Autodesk Fusion 360 part; units mm, degrees
note: some values were not read from the file. Chosen so that the rebuilt part matches the saved one: which face or edge a step refers to. Set by a fixed rule: which sketch regions a step uses.
(part 3 of 3)
sketch "SecondHoles" plane through (0, 0, 0) normal (0, 0, 1) x (1, 0, 0)
  circle A0 centre (-16.518, 39.156) radius 0.5
  arc A1 (-17.021, 38.656) -> (-17.021, 39.656) centre (-17.018, 39.156) ccw
  circle A2 centre (-16.518, 36.656) radius 0.5
  circle A3 centre (-17.018, 36.656) radius 0.5
  circle A4 centre (-16.518, 34.156) radius 0.5
  circle A5 centre (-17.018, 34.156) radius 0.5
  circle A6 centre (-16.518, 31.656) radius 0.5
  circle A7 centre (-16.518, 29.156) radius 0.5
  arc A8 (-17.021, 28.656) -> (-17.021, 29.656) centre (-17.018, 29.156) ccw
  circle A9 centre (-16.518, 26.656) radius 0.5
  arc A10 (-16.718, 26.256) -> (-16.718, 27.056) centre (-17.018, 26.656) ccw
  circle A11 centre (-16.518, 24.156) radius 0.5
  arc A12 (-17.021, 23.656) -> (-17.021, 24.656) centre (-17.018, 24.156) ccw
  circle A13 centre (-16.518, 21.656) radius 0.5
  circle A14 centre (-16.518, 19.156) radius 0.5
  arc A15 (-17.021, 18.656) -> (-17.021, 19.656) centre (-17.018, 19.156) ccw
  circle A16 centre (-16.518, 16.656) radius 0.5
  circle A17 centre (-17.018, 16.656) radius 0.5
  circle A18 centre (-16.518, 14.156) radius 0.5
  circle A19 centre (-17.018, 14.156) radius 0.5
  circle A20 centre (-16.518, 11.656) radius 0.5
  circle A21 centre (-17.018, 11.656) radius 0.5
  circle A22 centre (-16.518, 9.156) radius 0.5
  circle A23 centre (-17.018, 9.156) radius 0.5
  circle A24 centre (-16.518, 6.656) radius 0.5
  circle A25 centre (-17.018, 6.656) radius 0.5
  circle A26 centre (-16.518, 4.156) radius 0.5
  circle A27 centre (-17.018, 4.156) radius 0.5
  circle A28 centre (-2.024, 4.156) radius 0.5
  circle A29 centre (-1.524, 4.156) radius 0.5
  circle A30 centre (-2.024, 6.656) radius 0.5
  circle A31 centre (-2.024, 9.156) radius 0.5
  circle A32 centre (-2.024, 11.656) radius 0.5
  arc A33 (-1.524, 12.156) -> (-1.524, 11.156) centre (-1.524, 11.656) ccw
  circle A34 centre (-2.024, 14.156) radius 0.5
  arc A35 (-1.824, 14.556) -> (-1.824, 13.756) centre (-1.524, 14.156) ccw
  circle A36 centre (-2.024, 16.6514) radius 0.5
  arc A37 (-1.8277, 17.0532) -> (-1.8203, 16.2532) centre (-1.524, 16.656) ccw
  circle A38 centre (-2.024, 19.156) radius 0.5
  arc A39 (-1.824, 19.556) -> (-1.824, 18.756) centre (-1.524, 19.156) ccw
  circle A40 centre (-2.024, 21.656) radius 0.5
  arc A41 (-1.521, 22.156) -> (-1.521, 21.156) centre (-1.524, 21.656) ccw
  circle A42 centre (-2.024, 24.156) radius 0.5
  arc A43 (-1.824, 24.556) -> (-1.824, 23.756) centre (-1.524, 24.156) ccw
  circle A44 centre (-2.024, 26.656) radius 0.5
  arc A45 (-1.521, 27.156) -> (-1.521, 26.156) centre (-1.524, 26.656) ccw
  circle A46 centre (-2.024, 29.156) radius 0.503
  circle A47 centre (-2.024, 31.656) radius 0.503
  circle A48 centre (-2.024, 34.156) radius 0.5
  arc A49 (-1.824, 34.556) -> (-1.824, 33.756) centre (-1.524, 34.156) ccw
  circle A50 centre (-2.024, 36.656) radius 0.5
  arc A51 (-1.521, 37.156) -> (-1.521, 36.156) centre (-1.524, 36.656) ccw
  circle A52 centre (-2.024, 39.156) radius 0.5
  arc A53 (-1.824, 39.556) -> (-1.824, 38.756) centre (-1.524, 39.156) ccw
  circle A54 centre (-17.518, 39.156) radius 0.5
  circle A55 centre (-17.518, 36.656) radius 0.5
  circle A56 centre (-17.518, 34.156) radius 0.5
  circle A57 centre (-17.518, 31.656) radius 0.5
  circle A58 centre (-17.518, 29.156) radius 0.5
  circle A59 centre (-17.518, 26.656) radius 0.5
  circle A60 centre (-17.518, 24.156) radius 0.5
  arc A61 (-17.021, 24.656) -> (-17.021, 23.656) centre (-17.018, 24.156) ccw
  circle A62 centre (-17.518, 21.656) radius 0.5
  circle A63 centre (-17.518, 19.156) radius 0.5
  circle A64 centre (-17.518, 16.656) radius 0.5
  circle A65 centre (-17.518, 14.156) radius 0.5
  circle A66 centre (-17.518, 11.656) radius 0.5
  arc A67 (-17.318, 12.056) -> (-17.318, 11.256) centre (-17.018, 11.656) ccw
  circle A68 centre (-17.518, 9.156) radius 0.5
  circle A69 centre (-17.518, 6.656) radius 0.5
  arc A70 (-17.318, 7.056) -> (-17.318, 6.256) centre (-17.018, 6.656) ccw
  circle A71 centre (-17.5948, 4.156) radius 0.5768
  circle A72 centre (-1.0241, 4.1682) radius 0.5
  circle A73 centre (-1.024, 6.656) radius 0.5
  circle A74 centre (-1.524, 6.656) radius 0.5
  circle A75 centre (-1.024, 9.156) radius 0.5
  circle A76 centre (-1.524, 9.156) radius 0.5
  circle A77 centre (-1.024, 11.656) radius 0.5
  arc A78 (-1.524, 11.156) -> (-1.524, 12.156) centre (-1.524, 11.656) ccw
  circle A79 centre (-1.024, 14.156) radius 0.5
  circle A80 centre (-1.524, 14.156) radius 0.5
  circle A81 centre (-1.024, 16.6606) radius 0.5
  arc A82 (-1.8203, 16.2532) -> (-1.8277, 17.0532) centre (-1.524, 16.656) ccw
  circle A83 centre (-1.024, 19.156) radius 0.5
  circle A84 centre (-1.024, 21.656) radius 0.5
  circle A85 centre (-1.024, 24.156) radius 0.5
  circle A86 centre (-1.024, 26.656) radius 0.5
  circle A87 centre (-1.024, 29.156) radius 0.5
  circle A88 centre (-1.024, 31.656) radius 0.5
  circle A89 centre (-1.024, 34.1563) radius 0.5
  arc A90 (-1.2237, 33.7562) -> (-1.2243, 34.5562) centre (-1.524, 34.156) ccw
  circle A91 centre (-1.024, 36.656) radius 0.5
  arc A92 (-1.521, 36.156) -> (-1.521, 37.156) centre (-1.524, 36.656) ccw
  circle A93 centre (-1.024, 39.156) radius 0.5
  circle A94 centre (-17.018, 31.656) radius 0.5
  circle A95 centre (-17.018, 21.656) radius 0.5
  circle A96 centre (-1.524, 19.156) radius 0.5
  circle A97 centre (-1.524, 21.656) radius 0.5
  circle A98 centre (-1.524, 24.156) radius 0.5
  circle A99 centre (-1.524, 26.656) radius 0.5
  circle A100 centre (-1.524, 29.156) radius 0.5
  circle A101 centre (-1.524, 31.656) radius 0.5
  circle A102 centre (-1.524, 39.156) radius 0.5
  arc A103 (-17.021, 39.656) -> (-17.021, 38.656) centre (-17.018, 39.156) ccw
  point P0 (-2.024, 4.156)
  point P1 (-2.024, 6.656)
  point P2 (-2.024, 9.156)
  point P3 (-17.518, 36.656)
  point P4 (-17.518, 34.156)
  point P5 (-17.518, 16.656)
  point P6 (-17.518, 14.156)
  point P7 (-17.518, 9.156)
  point P8 (-2.024, 19.156)
  point P9 (-2.024, 29.156)
  point P10 (-2.024, 31.656)
  point P11 (-17.518, 39.156)
  point P12 (-17.518, 31.656)
  point P13 (-17.518, 29.156)
  point P14 (-17.518, 26.656)
  point P15 (-17.518, 21.656)
  point P16 (-17.518, 19.156)
  constraint midpoint A0.centre A1
  constraint coincident A0 A1.centre
  constraint coincident A2.centre A3
  constraint coincident A2 A3.centre
  constraint coincident A4.centre A5
  constraint coincident A4 A5.centre
  constraint coincident A6.centre A94
  constraint coincident A6 A94.centre
  constraint midpoint A7.centre A8
  constraint coincident A7 A8.centre
  constraint midpoint A9.centre A10
  constraint coincident A9 A10.centre
  constraint midpoint A11.centre A12
  constraint coincident A11 A12.centre
  constraint coincident A13.centre A95
  constraint coincident A13 A95.centre
  constraint midpoint A14.centre A15
  constraint coincident A14 A15.centre
  constraint coincident A16.centre A17
  constraint coincident A16 A17.centre
  constraint coincident A18.centre A19
  constraint coincident A18 A19.centre
  constraint coincident A20.centre A21
  constraint coincident A20 A21.centre
  constraint coincident A22.centre A23
  constraint coincident A22 A23.centre
  constraint coincident A24.centre A25
  constraint coincident A24 A25.centre
  constraint coincident A26.centre A27
  constraint coincident A26 A27.centre
  constraint coincident P0 A28.centre
  constraint coincident A28 A29.centre
  constraint coincident P1 A30.centre
  constraint coincident P2 A31.centre
  constraint midpoint A32.centre A33
  constraint coincident A32 A33.centre
  constraint midpoint A34.centre A35
  constraint coincident A34 A35.centre
  constraint midpoint A36.centre A37
  constraint coincident A36 A37.centre
  constraint coincident A38 A39.centre
  constraint midpoint A40.centre A41
  constraint coincident A40 A41.centre
  constraint midpoint A42.centre A43
  constraint midpoint A44.centre A45
  constraint coincident A44 A45.centre
  constraint midpoint A48.centre A49
  constraint coincident A48 A49.centre
  constraint midpoint A50.centre A51
  constraint coincident A50 A51.centre
  constraint midpoint A52.centre A53
  constraint coincident A52 A53.centre
  constraint coincident A54 A1.centre
  constraint coincident P3 A55.centre
  constraint coincident A3.centre A55
  constraint tangent A2 A55
  constraint coincident P4 A56.centre
  constraint coincident A5.centre A56
  constraint tangent A4 A56
  constraint coincident A57 A94.centre
  constraint tangent A6 A57
  constraint coincident A8.centre A58
  constraint coincident A10.centre A59
  constraint midpoint A60.centre A61
  constraint coincident A12.centre A60
  constraint coincident A62 A95.centre
  constraint tangent A13 A62
  constraint coincident A15.centre A63
  constraint coincident P5 A64.centre
  constraint coincident A17.centre A64
  constraint tangent A16 A64
  constraint coincident P6 A65.centre
  constraint coincident A19.centre A65
  constraint tangent A18 A65
  constraint midpoint A66.centre A67
  constraint coincident A21.centre A66
  constraint tangent A20 A66
  constraint coincident P7 A68.centre
  constraint coincident A23.centre A68
  constraint tangent A22 A68
  constraint midpoint A69.centre A70
  constraint coincident A25.centre A69
  constraint tangent A24 A69
  constraint coincident A27.centre A71
  constraint tangent A26 A71
  constraint coincident A29 A72.centre
  constraint coincident A29.centre A72
  constraint coincident A73.centre A74
  constraint coincident A73 A74.centre
  constraint tangent A30 A73
  constraint coincident A75.centre A76
  constraint coincident A75 A76.centre
  constraint tangent A31 A75
  constraint midpoint A77.centre A78
  constraint coincident A33.centre A77
  constraint coincident A79.centre A80
  constraint coincident A35.centre A79
  constraint tangent A34 A79
  constraint midpoint A81.centre A82
  constraint coincident A37.centre A81
  constraint coincident A83.centre A96
  constraint coincident A39.centre A83
  constraint tangent A38 A83
  constraint coincident A84.centre A97
  constraint coincident A41.centre A84
  constraint coincident A85.centre A98
  constraint coincident A43.centre A85
  constraint tangent A42 A85
  constraint coincident A86.centre A99
  constraint coincident A45.centre A86
  constraint tangent A44 A86
  constraint coincident A87.centre A100
  constraint coincident A87 A100.centre
  constraint coincident A88.centre A101
  constraint coincident A88 A101.centre
  constraint midpoint A89.centre A90
  constraint coincident A49.centre A89
  constraint midpoint A91.centre A92
  constraint coincident A51.centre A91
  constraint coincident A93.centre A102
  constraint coincident A53.centre A93
extrude "Extrude54" cut sketch "SecondHoles" against normal blind 9 contours A0 A1 | A0 A1 | A0 A1 A54 A103 | A0 A1 A54 A103 | A54 A103 | A2 A3 | A2 A3 | A4 A5 | A4 A5 | A6 A94 | A6 A94 | A7 A8 | A7 A8 | A9 | A11 A12 | A11 A12 | A13 A95 | A13 A95 | A14 A15 | A14 A15 | A16 A17 | A16 A17 | A18 A19 | A18 A19 | A20 A21 | A20 A21 | A22 A23 | A22 A23 | A24 A25 | A24 A25 | A26 A27 | A26 A27 | A28 A29 | A28 A29 | A30 A74 | A30 A74 | A31 A76 | A31 A76 | A32 A33 | A32 A33 | A34 A35 A80 | A34 A35 A80 | A36 A37 A82 | A36 A37 A82 | A38 A39 A96 | A38 A39 A96 | A40 A41 A97 | A40 A41 A97 | A42 A43 A98 | A42 A43 A98 | A44 A45 A99 | A44 A45 A99 | A46 A87 | A46 A87 A100 | A46 A100 | A47 A88 | A47 A88 A101 | A47 A101 | A48 | A50 A51 | A50 A51 | A52 A53 A102 | A52 A53 A102 picked at (-17.3495, 39.1311) picked at (-1.6898, 29.081) picked at (-1.6898, 31.581) bodies 1
extrude "Extrude57" cut sketch "SecondHoles" against normal blind 9 contours A0 A1 | A0 A1 | A0 A1 A54 A103 | A0 A1 A54 A103 | A54 A103 | A54 A103 | A2 A3 | A2 A3 | A2 A3 A55 | A2 A3 A55 | A3 A55 | A3 A55 | A4 A5 | A4 A5 | A4 A5 A56 | A4 A5 A56 | A5 A56 | A5 A56 | A6 A94 | A6 A94 | A6 A57 A94 | A6 A57 A94 | A57 A94 | A57 A94 | A7 A8 | A58 | A7 A8 | A9 | A59 | A11 A12 | A11 A12 | A11 A12 A60 A61 | A11 A12 A60 A61 | A60 A61 | A60 A61 | A13 A95 | A13 A95 | A13 A62 A95 | A13 A62 A95 | A62 A95 | A62 A95 | A14 A15 | A63 | A14 A15 | A16 A17 | A16 A17 | A16 A17 A64 | A16 A17 A64 | A17 A64 | A17 A64 | A18 A19 | A18 A19 | A18 A19 A65 | A18 A19 A65 | A19 A65 | A19 A65 | A20 A21 | A20 A21 | A20 A21 A66 | A20 A21 A66 | A21 A66 A67 | A21 A66 A67 | A22 A23 | A22 A23 | A22 A23 A68 | A22 A23 A68 | A23 A68 | A23 A68 | A24 A25 | A24 A25 | A24 A25 A69 | A24 A25 A69 | A25 A69 A70 | A25 A69 A70 | A26 A27 | A26 A27 | A26 A27 A71 | A26 A27 A71 | A27 A71 | A27 A71 | A28 A29 | A28 A29 A72 | A28 A29 A72 | A28 A29 | A29 A72 | A30 A74 | A30 A73 A74 | A30 A73 A74 | A73 A74 | A30 A74 | A73 A74 | A31 A76 | A31 A75 A76 | A31 A75 A76 | A75 A76 | A31 A76 | A75 A76 | A32 A33 | A32 A33 A77 A78 | A32 A33 A77 A78 | A77 A78 | A32 A33 | A77 A78 | A34 A35 A80 | A34 A79 A80 | A34 A79 A80 | A79 A80 | A34 A35 A80 | A79 A80 | A36 A37 A82 | A36 A81 A82 | A36 A81 A82 | A81 A82 | A36 A37 A82 | A81 A82 | A38 A39 A96 | A38 A83 A96 | A38 A83 A96 | A83 A96 | A38 A39 A96 | A83 A96 | A40 A41 A97 | A40 A41 A84 A97 | A40 A41 A84 A97 | A84 A97 | A40 A41 A97 | A84 A97 | A42 A43 A98 | A42 A85 A98 | A42 A85 A98 | A85 A98 | A42 A43 A98 | A85 A98 | A44 A45 A99 | A44 A45 A86 A99 | A44 A45 A86 A99 | A86 A99 | A44 A45 A99 | A86 A99 | A46 A87 | A46 A87 A100 | A46 A87 A100 | A46 A87 A100 | A46 A87 A100 | A46 A100 | A87 A100 | A47 A88 | A47 A88 A101 | A47 A88 A101 | A47 A88 A101 | A47 A88 A101 | A47 A101 | A88 A101 | A48 | A89 | A50 A51 | A50 A51 A91 A92 | A50 A51 A91 A92 | A91 A92 | A50 A51 | A91 A92 | A52 A53 A102 | A52 A93 A102 | A52 A93 A102 | A93 A102 | A52 A53 A102 | A93 A102 picked at (-0.6926, 4.1396) bodies 1
extrude "Extrude55" cut sketch "Sketch14" against normal blind 6.15 contours L77 A25 L78 A26 L115 L116 L118 L119 L178 | A26 L115 L116 L118 L119 L178 | A3 L170 L171 L172 L173 L188 | L25 A3 L26 A4 L170 L171 L172 L173 L188 | L52 A11 L53 A12 L121 L122 L124 L125 L179 | A11 L121 L122 L124 L125 L179 | L55 A13 L56 A14 L127 L128 L130 L131 L180 | A13 L127 L128 L130 L131 L180 | L30 A5 L31 A6 L166 L167 L168 L169 L187 | A5 L166 L167 L168 L169 L187 | L33 A7 L34 A8 L162 L163 L164 L165 L186 | A7 L162 L163 L164 L165 L186 | L37 A9 L38 A10 L156 L157 L160 L161 L185 | A9 L156 L157 L160 L161 L185 | L58 A15 L59 A16 L132 L133 L134 L135 L181 | A15 L132 L133 L134 L135 L181 | L61 A17 L62 A18 L136 L137 L138 L139 L182 | A17 L136 L137 L138 L139 L182 | L65 A19 L66 A20 L85 L86 L100 | A20 L85 L86 L100 | L68 A21 L69 A22 L142 L143 L146 L147 L183 | A22 L142 L143 L146 L147 L183 | L74 A23 L75 A24 L174 L175 L176 L177 L189 | A24 L174 L175 L176 L177 L189 | L81 A27 L82 A28 L149 L150 L152 L153 L184 | A27 L149 L150 L152 L153 L184 bodies 1
extrude "Extrude56" cut sketch "BluetoothFacade" against normal blind 6.1 contours L42 L43 L44 L45 L87 L89 | L47 L49 L88 L89 | L28 L29 L31 L32 L87 L90 | L35 L39 L87 L90 bodies 1
move_body "Move34" bodies 1 to x (1, 0, 0) y (0, 1, 0) z (0, 0, 1) at (0, 0, 9)
extrude "Extrude58" cut sketch "Sketch14" along normal blind 3.5 contours L7 L114 L115 L117 L207 | A26 L115 L117 L118 L207 | A26 L115 L116 L118 L119 L178 | L9 L170 L172 L206 | A3 L170 L172 L206 | A3 L170 L171 L172 L173 L188 | L10 L120 L121 L123 L207 | A11 L121 L123 L124 L207 | A11 L121 L122 L124 L125 L179 | L11 L126 L129 L207 | A13 L126 L127 L129 L130 L207 | A13 L127 L128 L130 L131 L180 | A0 | A0 L195 L197 A30 | L195 A30 L206 | L197 A30 L206 | A29 L194 L195 L196 L197 L206 | A29 L92 | A29 L92 | A1 | A1 L199 L201 A32 | L199 L207 A32 | L201 L207 A32 | L90 L198 L199 L200 L201 L207 | A2 | A2 L203 L205 A31 | L203 A31 L207 | L205 A31 L207 | L91 L202 L203 L204 L205 L207 | A5 L166 L167 L168 L169 L187 | A5 L166 L168 L206 | L101 L166 L168 L206 | A7 L162 L163 L164 L165 L186 | A7 L162 L164 L206 | L94 L162 L164 L206 | A9 L156 L157 L160 L161 L185 | A9 L154 L155 L156 L158 L159 L160 L206 | L154 L158 L190 L206 | A15 L132 L133 L134 L135 L181 | A15 L132 L134 L207 | L96 L132 L134 L207 | A17 L136 L137 L138 L139 L182 | A17 L136 L138 L207 | L97 L136 L138 L207 | A20 L85 L86 L99 | A20 L85 L86 L100 | A22 L140 L141 L142 L144 L145 L146 L207 | A22 L142 L143 L146 L147 L183 | L98 L140 L144 L207 | A24 L174 L176 L206 | A24 L174 L175 L176 L177 L189 | L95 L174 L176 L206 | A27 L149 L150 L152 L153 L184 | A27 L93 L148 L149 L151 L152 picked at (-21.3171, 24.4597) picked at (2.6582, 26.2398) picked at (2.799, 21.3024) bodies 1
move_body "Move35" bodies 1 to x (1, 0, 0) y (0, 1, 0) z (0, 0, 1) at (0, 0, -9)
extrude "Extrude59" cut sketch "BluetoothFacade" against normal blind 5.5 contours L14 L44 L46 L75 A15 A17 L79 L87 | L14 L31 L42 L78 A17 A19 L82 L87 | L14 L28 L38 L39 L81 A19 A21 L85 L87 bodies 1
extrude "Extrude60" cut sketch "Sketch14" against normal blind 9 contours A0 | A1 | A2 bodies 1
extrude "Extrude61" cut sketch "Sketch14" against normal blind 6 contours A0 | A0 L195 L197 A30 | A0 L195 L197 A30 | A1 | A1 L199 L201 A32 | A1 L199 L201 A32 | A2 | A2 L203 L205 A31 | A2 L203 L205 A31 bodies 1
hidden bodies 10 11
equation "SmallBitSize = 0.8 mm"
equation "HalfSmallBitSize = SmallBitSize / 2"
equation "d27 = HalfSmallBitSize"
equation "d28 = -HalfSmallBitSize"
equation "d29 = HalfSmallBitSize"
equation "d30 = -HalfSmallBitSize"
equation "d31 = HalfSmallBitSize"
equation "d32 = HalfSmallBitSize"
equation "d33 = HalfSmallBitSize"
equation "d34 = HalfSmallBitSize"
equation "d35 = HalfSmallBitSize"
equation "d36 = HalfSmallBitSize"
equation "d39 = -HalfSmallBitSize"
equation "d40 = -HalfSmallBitSize"
equation "d41 = -HalfSmallBitSize"
equation "d42 = -HalfSmallBitSize"
equation "d43 = -HalfSmallBitSize"
equation "d44 = -HalfSmallBitSize"
equation "d45 = WoodHeight"
equation "WoodHeight = 9 mm"
equation "d48 = WoodHeight"
equation "d50 = -SpaceForResistance - NanoPlasticPinProtection - NanoSurfaceHeight"
equation "d56 = WoodHeight"
equation "d61 = -WoodHeight"
equation "d62 = -NanoSurfaceHeight - NanoPlasticPinProtection"
equation "d64 = -NanoSurfaceHeight - NanoPlasticPinProtection"
equation "d70 = WoodHeight"
equation "JoinSize = 3.1 mm"
equation "d228 = -HalfSmallBitSize"
equation "d232 = WoodHeight"
equation "HolesBorder = SmallBitSize + 0.5 mm"
equation "d327 = SmallBitSize"
equation "d328 = SmallBitSize"
equation "d329 = SmallBitSize"
equation "d330 = SmallBitSize"
equation "d335 = SmallBitSize"
equation "d336 = HalfSmallBitSize"
equation "d337 = -HalfSmallBitSize"
equation "d338 = HalfSmallBitSize"
equation "d339 = -HalfSmallBitSize"
equation "d340 = HalfSmallBitSize"
equation "d341 = -HalfSmallBitSize"
equation "d342 = HalfSmallBitSize"
equation "d343 = -HalfSmallBitSize"
equation "d346 = -WoodHeight"
equation "d353 = HalfSmallBitSize"
equation "d354 = -HalfSmallBitSize"
equation "d355 = HalfSmallBitSize"
equation "d356 = -HalfSmallBitSize"
equation "d394 = -WoodHeight"
equation "d405 = HalfMiddleBitSize"
equation "d406 = HalfMiddleBitSize"
equation "d407 = HalfMiddleBitSize"
equation "d408 = HalfMiddleBitSize * -1"
equation "d409 = HalfMiddleBitSize * -1"
equation "d410 = HalfMiddleBitSize * -1"
equation "d436 = WoodHeight"
equation "d446 = -TopDepthTunnels"
equation "TopDepthTunnels = 6 mm"
equation "d451 = -TopDepthTunnels - 1 mm"
equation "d453 = -WoodHeight"
equation "d455 = -WoodHeight"
equation "d457 = -WoodHeight"
equation "NanoSurfaceHeight = 2.1 mm"
equation "NanoPlasticPinProtection = 2 mm"
equation "d461 = -NanoSurfaceHeight"
equation "d467 = -TopDepthTunnels"
equation "d472 = WoodHeight"
equation "d473 = WoodHeight - TopDepthTunnels + 3 mm"
equation "d477 = -WoodHeight"
equation "d478 = -TopDepthTunnels + 1 mm"
equation "d483 = -NanoSurfaceHeight"
equation "d486 = -NanoSurfaceHeight - NanoPlasticPinProtection"
equation "d488 = -WoodHeight"
equation "HalfMiddleBitSize = MiddleBitSize / 2"
equation "d491 = HalfMiddleBitSize * -1"
equation "d492 = HalfMiddleBitSize"
equation "MiddleBitSize = SmallBitSize"
equation "d496 = -TopDepthTunnels - 0.15 mm"
equation "d498 = -TopDepthTunnels - 0.1 mm"
equation "SpaceForResistance = 2.4 mm"
equation "d501 = -WoodHeight"
equation "d508 = SmallBitSize"
equation "d509 = SmallBitSize"
equation "d511 = SmallBitSize"
equation "d545 = WoodHeight"
equation "d546 = HalfSmallBitSize"
equation "d547 = HalfSmallBitSize"
equation "d548 = HalfSmallBitSize"
equation "d550 = HalfSmallBitSize"
equation "d551 = HalfSmallBitSize"
equation "d552 = HalfSmallBitSize"
equation "d553 = HalfSmallBitSize"
equation "d554 = HalfSmallBitSize"
equation "d555 = -HalfSmallBitSize"
equation "d556 = -HalfSmallBitSize"
equation "d557 = -HalfSmallBitSize"
equation "d558 = -HalfSmallBitSize"
equation "d559 = -HalfSmallBitSize"
equation "d561 = -HalfSmallBitSize"
equation "d562 = -HalfSmallBitSize"
equation "d563 = -HalfSmallBitSize"
equation "d564 = -HalfSmallBitSize"
equation "d565 = -HalfSmallBitSize"
equation "d566 = -HalfSmallBitSize"
equation "d567 = -HalfSmallBitSize * -1"
equation "d568 = -HalfSmallBitSize * -1"
equation "d569 = -HalfSmallBitSize * -1"
equation "d570 = WoodHeight - TopDepthTunnels + 0.5 mm"
equation "d575 = -HalfSmallBitSize * -1"
equation "d576 = -HalfSmallBitSize"
equation "d577 = -HalfSmallBitSize * -1"
equation "d578 = -HalfSmallBitSize"
equation "d581 = WoodHeight"
equation "d584 = -WoodHeight"
equation "d585 = -TopDepthTunnels + 0.5 mm"
equation "d587 = -WoodHeight"
equation "d589 = -TopDepthTunnels"
named bodies: "WoodAdaptator", "CapacitivePinJoin", "BluetoothBatteryPinJoin"
